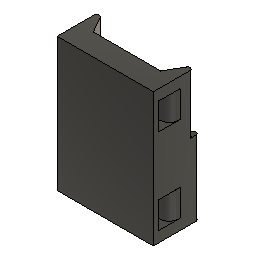
XIDIBEI Transducer Holder v5 (Autodesk Fusion 360 design; units mm, degrees)
Autodesk Fusion 360 part; units mm, degrees
sketch "Sketch1" plane through (0, 0, 0) normal (0, 0, 1) x (1, 0, 0)
  circle A0 centre (0, 0) radius 10.5
  line L0 (-6.3076, 10.925) -> (-12.6151, 0)
  line L1 (-12.6151, 0) -> (-6.3076, -10.925)
  line L2 (-6.3076, -10.925) -> (6.3076, -10.925)
  line L3 (6.3076, -10.925) -> (12.6151, 0)
  line L4 (12.6151, 0) -> (6.3076, 10.925)
  line L5 (6.3076, 10.925) -> (-6.3076, 10.925)
  line L6 (-4.6188, 8) -> (-9.2376, 0)
  line L7 (-9.2376, 0) -> (-4.6188, -8)
  line L8 (-4.6188, -8) -> (4.6188, -8)
  line L9 (4.6188, -8) -> (9.2376, 0)
  line L10 (9.2376, 0) -> (4.6188, 8)
  line L11 (4.6188, 8) -> (-4.6188, 8)
  dimension "d2" = 21
  dimension "d3" = 10.925
  dimension "d15" = 8
  constraint coincident A0.centre origin
  measures "d2" diameter of A0
  measures "d3" distance of A0.centre L5
  measures "d15" distance of A0.centre L11
extrude "Extrude2" add sketch "Sketch1" along normal blind 15 contours A0 | L6 L7 L8 L9 L10 L11 makes body 1
extrude "Extrude3" add sketch "Sketch1" along normal blind 12 from surface at 15 contours A0 | L0 L1 L2 L3 L4 L5 | L6 L7 L8 L9 L10 L11 bodies 1
extrude "Extrude4" add sketch "Sketch1" along normal blind 17 from surface at 27 contours L6 L7 L8 L9 L10 L11 bodies 1
sketch "Sketch2" plane through (0, 0, 0) normal (0, 1, 0) x (1, 0, 0)
  line L0 (-9, -1) -> (9, -1)
  line L1 (9, -1) -> (9, -26)
  line L2 (9, -26) -> (-9, -26)
  line L3 (-9, -26) -> (-9, -1)
  constraint horizontal L0
  constraint vertical L1
  constraint horizontal L2
  constraint vertical L3
extrude "Extrude5" add sketch "Sketch2" against normal blind 15 separate body makes body 2
combine "Combine1" operation cut target body 2 tool bodies 1 keep tools
sketch "Sketch3" plane through (9, 0, 0) normal (1, 0, 0) x (0, 1, 0)
  line L0 (-6.2615, 15) -> (-6.2615, 26)
  line L1 (-6.2615, 26) -> (-15, 26)
  line L2 (-15, 26) -> (-15, 1)
  line L3 (-15, 1) -> (-5.4083, 1)
  line L4 (-5.4083, 1) -> (-5.4083, 15)
  line L5 (-5.4083, 15) -> (-6.2615, 15)
  line L6 (-14, 24) -> (-12, 24)
  line L7 (-12, 24) -> (-12, 19)
  line L8 (-12, 19) -> (-14, 19)
  line L9 (-14, 19) -> (-14, 24)
  line L10 (-14, 3) -> (-12, 3)
  line L11 (-12, 3) -> (-12, 8)
  line L12 (-12, 8) -> (-14, 8)
  line L13 (-14, 8) -> (-14, 3)
  dimension "d24" = 2
  dimension "d25" = 5
  dimension "d26" = 2
  dimension "d27" = 5
  dimension "d28" = 2
  dimension "d29" = 2
  constraint horizontal L6
  constraint vertical L7
  constraint horizontal L8
  constraint vertical L9
  constraint horizontal L10
  constraint vertical L11
  constraint horizontal L12
  constraint vertical L13
  measures "d24" distance of L1 L6
  measures "d25" distance of L6.start L8.end
  measures "d26" distance of L3 L10
  measures "d27" distance of L10.start L12.end
  measures "d28" distance of L7 L9
  measures "d29" distance of L11 L13
extrude "Extrude6" cut sketch "Sketch3" against normal blind 28 contours L6 L7 L8 L9 | L10 L11 L12 L13 bodies 2
fillet "Fillet1" radius 2 curvature continuous 4 edges at (9, -12, 21.5) (9, -12, 5.5) (-9, -12, 21.5) (-9, -12, 5.5) on bodies 2
fillet "Fillet2" radius 0.5 4 edges at (-9, -5.4083, 8) (-9, -6.2615, 20.5) (9, -6.2615, 20.5) (9, -5.4083, 8) on bodies 2
hidden bodies 1
equation "d3 = 21.85 mm / 2"
equation "d26 = d24"
equation "d27 = d25"
equation "d28 = d24"
equation "d29 = d24"
